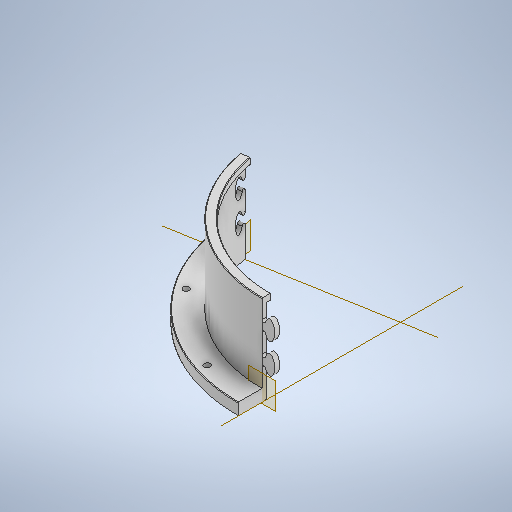
# Autodesk Inventor part: Cylinder Segment_01_PuzzlePiece_Q2+4
Saved by Autodesk Inventor 2025 (Build 290162000, 162)
## iProperties
Created: 2024-04-11
Part Number: Cylinder Segment_01_PuzzlePiece_Q2+4
Material: Generic
Document SubType Name: Modeling
Designer: Thienan Hoang
Density: 1 g/cm^3
Appearance: Default
Author: Thienan Hoang
Autodesk Inventor part; units mm, degrees
ref_plane "YZ Plane" through (0, 0, 0) normal (1, 0, 0) x (0, 1, 0)
ref_plane "XZ Plane" through (0, 0, 0) normal (0, 1, 0) x (-1, 0, 0)
ref_plane "XY Plane" through (0, 0, 0) normal (0, 0, 1) x (1, 0, 0)
sketch "Sketch1" plane through (0, 0, 0) normal (0, 1, 0) x (-1, 0, 0)
  circle A0 centre (0, 0) radius 135
  circle A1 centre (0, 0) radius 115
  circle A2 centre (0, 0) radius 111.375
  circle A3 centre (0, 0) radius 9.5
  dimension "Absolute_Diameter" = 270
  dimension "Diameter_No_Outer_Lip" = 230
  dimension "Inner_Cylinder_Diameter" = 222.75
  dimension "Lip_Diameter" = 19
  constraints: 4 centre point, 4 coincident
  measures "Absolute_Diameter" diameter of A0
  measures "Diameter_No_Outer_Lip" diameter of A1
  measures "Inner_Cylinder_Diameter" diameter of A2
  measures "Lip_Diameter" diameter of A3
extrude "Extrusion1" add sketch "Sketch1" along normal blind 10 contours A0
extrude "Extrusion2" add sketch "Sketch1" along normal blind 75 contours A1
sketch "Sketch2" plane through (0, 75, 0) normal (0, 1, 0) x (1, 0, 0)
  circle A0 centre (0, 0) radius 115
  circle A1 centre (0, 0) radius 107.75
  dimension "Lip_Hang" = 7.25
  dimension "Lip_Diameter_Out" = 230
  dimension "Inner_Lip_Diameter" = 215.5
  constraints: 2 centre point, 1 coincident
  measures "Lip_Hang" radial gap between concentric circles of A0 A1
  measures "Lip_Diameter_Out" diameter of A0
  measures "Inner_Lip_Diameter" diameter of A1
extrude "Extrusion7" add sketch "Sketch2" against normal blind 5
chamfer "Chamfer1" distance 0.5 angle 45 2 edges at (115, 75, 0) (-107.75, 75, 0)
chamfer "Chamfer2" distance 0.5 angle 45 3 edges at (135, 10, 0) (135, 0, 0) (111.375, 0, 0)
sketch "Sketch3" plane through (0, 10, 0) normal (0, 1, 0) x (1, 0, 0)
  circle A0 centre (0, 0) radius 127.5
  circle A1 centre (-127.5, 0) radius 2.5
  circle A2 centre (-103.1497, -74.9426) radius 2.5
  circle A3 centre (-39.3997, -121.2597) radius 2.5
  circle A4 centre (39.3997, -121.2597) radius 2.5
  circle A5 centre (103.1497, -74.9426) radius 2.5
  circle A6 centre (127.5, 0) radius 2.5
  circle A7 centre (103.1497, 74.9426) radius 2.5
  circle A8 centre (39.3997, 121.2597) radius 2.5
  circle A9 centre (-39.3997, 121.2597) radius 2.5
  circle A10 centre (-103.1497, 74.9426) radius 2.5
  dimension "d27" = 255
  dimension "d28" = 5
  dimension "d31" = 360
  constraints: 10 centre point, 1 coincident, 1 horizontal alignment, 23 other
  measures "d28" diameter of A1
extrude "Extrusion8" cut sketch "Sketch3" against normal blind 10 contours A0 A6 | A0 A6 | A7 A0 | A0 A7 | A5 A0 | A0 A5 | A8 A0 | A0 A8 | A4 A0 | A0 A4 | A9 A0 | A0 A9 | A3 A0 | A0 A3 | A10 A0 | A0 A10 | A2 A0 | A0 A2 | A1 A0 | A0 A1
sketch "Sketch5" plane through (0, 0, 0) normal (0, -1, 0) x (1, 0, 0)
  circle A0 centre (0, 0) radius 135 projected
  line L0 (0, 135) -> (0, -135)
  line L1 (-148.9093, 26.2567) -> (158.1235, -27.8814)
  point P0 (-132.949, 23.4425)
  point P1 (132.949, -23.4425)
  dimension "d48" = 80
  constraints: 4 end point, 2 point on circle, 1 midpoint, 1 point on line, 1 vertical
  measures "d48" angle of L0 L1
extrude "Quadrant Cut" cut sketch "Sketch5" against normal through all contours A0 L1 L0 | A0 L0 L1 | L1 L0 A0 picked at (89.6719, 5.4242) picked at (5.2242, -89.6957) picked at (-5.2242, -89.6957)
ref_plane "Bm Plane" through (0, 10, 115) normal (0, 0, 1) x (1, 0, 0)
ref_plane "Work Plane2" through (-113.2529, 10, 19.9695) normal (0.9848078, 0, -0.1736482) x (0, 1, 0)
sketch "Sketch6" plane through (0, 10, 115) normal (0, 0, 1) x (1, 0, 0)
  ellipse E0 centre (6.3807, 45) end of major axis (6.3807, 53) minor radius 4 (2.9384, 40.9256) -> (2.9384, 49.0744) ccw
  line L0 (-13.5414, 32.5) -> (13.5791, 32.5) construction
  line L1 (-1.4334, 45) -> (1.8235, 45) construction
  line L2 (0, 51) -> (0, 65)
  line L3 (0, 0) -> (0, 64.5)
  arc A0 (0, 49.5) -> (2.9384, 49.0744) centre (1.5, 49.5) ccw
  arc A1 (2.9384, 40.9256) -> (0, 40.5) centre (1.5, 40.5) ccw
  line L4 (-1.4334, 20) -> (1.8235, 20) construction
  arc A2 (2.9384, 15.9256) -> (0, 15.5) centre (1.5, 15.5) ccw
  arc A3 (0, 24.5) -> (2.9384, 24.0744) centre (1.5, 24.5) ccw
  ellipse E1 centre (6.3807, 20) end of major axis (6.3807, 12) minor radius 4 (2.9384, 15.9256) -> (2.9384, 24.0744) ccw
  line L5 (-112.7605, 65) -> (0, 65) construction
  point P0 (0, -10)
  point P1 (0, 39)
  point P2 (0, 14)
  point P3 (0, 26)
  point P4 (0, 15.5)
  dimension "d51" = 8
  dimension "d52" = 4
  dimension "d53" = 3
  dimension "d54" = 4.5
  constraints: 13 symmetric about line, 10 end point, 8 point on circle, 4 centre point, 4 point on line, 1 horizontal, 1 tangent, 12 other
  measures "d53" diameter of A0
  measures "d54" distance from line of L1 A0.centre
extrude "Extrusion10" add sketch "Sketch6" against normal up to surface round surface about axis through (0, 0, 0) along (0, 1, 0) radius 111.375 far side no
sketch "Sketch7" plane through (-113.2529, 10, 19.9695) normal (0.9848078, 0, -0.1736482) x (0, 1, 0)
  ellipse E0 centre (45.019, 6.684) end of major axis (53.119, 6.684) minor radius 4.1 (49.0825, 3.1373) -> (40.9556, 3.1373) ccw
  line L0 (45.019, 6.684) -> (45.019, 0.4162) construction
  arc A0 (49.0825, 3.1373) -> (49.519, 0.1) centre (49.519, 1.65) ccw
  line L1 (64.5, 0) -> (0, 0)
  line L2 (65, 0.1) -> (0, 0.1)
  line L3 (-0.5, 0) -> (-9.5, 0)
  line L4 (49.519, 0.1) -> (-9.5, 0.1)
  line L5 (-9.5, 0.1) -> (-10, 0.1)
  arc A1 (40.519, 0.1) -> (40.9556, 3.1373) centre (40.519, 1.65) ccw
  line L6 (19.981, 6.684) -> (19.981, 0.4162) construction
  arc A2 (15.481, 0.1) -> (15.9175, 3.1373) centre (15.481, 1.65) ccw
  line L7 (0, 0.1) -> (65, 0.1)
  line L8 (0.5, 0) -> (65, 0)
  arc A3 (24.0444, 3.1373) -> (24.481, 0.1) centre (24.481, 1.65) ccw
  ellipse E1 centre (19.981, 6.684) end of major axis (11.881, 6.684) minor radius 4.1 (24.0444, 3.1373) -> (15.9175, 3.1373) ccw
  line L9 (65, 0) -> (64.5, 0)
  line L10 (0, 0) -> (-0.5, 0)
  line L11 (-9.5, 0) -> (-10, 0)
  line L12 (65, 0) -> (65, 0.1)
  line L13 (-10, 0) -> (-10, 0.1)
  line L14 (65, 0) -> (64.5, 0) projected
  point P0 (-10, 0)
  point P1 (32.5, -13.5778)
  point P2 (0.5, 0)
  point P3 (65, 0.1)
  point P4 (49.519, 0.1)
  point P5 (24.481, 0.1)
  point P6 (15.481, 0.1)
  dimension "d58" = 4.1
  dimension "d59" = 8.1
  dimension "d60" = 4.5
  dimension "d61" = 3.1
  dimension "d62" = 0.1
  dimension "d63" = 0.1
  constraints: 24 end point, 8 point on circle, 4 centre point, 2 vertical, 1 horizontal, 1 parallel, 1 point on line, 1 symmetric about line, 1 tangent, 16 other
  measures "d60" distance from line of L0 A0.centre
  measures "d61" diameter of A0
  measures "d62" distance of the line from the sketch origin of L2
  measures "d63" distance between parallel lines of L3 L4
extrude "Extrusion11" cut sketch "Sketch7" along normal through all both and the other way through all
body "Solid1"
